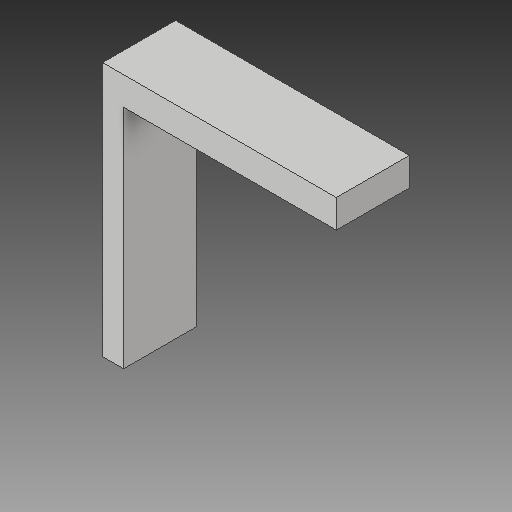
# Autodesk Inventor part: frame2
Saved by Autodesk Inventor 2019 (Build 230136000, 136)
## iProperties
Created: 2020-03-15
Part Number: frame2
Material: Generic
Document SubType Name: Modeling
Designer: Pulag
Mass: 4.15559 g
Surface Area: 27.541 cm^2
Volume: 4.15559 cm^3
Density: 1 g/cm^3
Appearance: Default
Author: Pulag
Autodesk Inventor part; units mm, degrees
ref_plane "YZ Plane" through (0, 0, 0) normal (1, 0, 0) x (0, 1, 0)
ref_plane "XZ Plane" through (0, 0, 0) normal (0, 1, 0) x (-1, 0, 0)
sketch "Sketch2" plane through (0, 0, 0) normal (0, 0, 1) x (1, 0, 0)
  line L0 (0.6059, 79.2071) -> (0.6059, 64.0071) projected
  line L1 (-21.8941, 64.0071) -> (-21.8941, 79.2071) projected
  line L2 (-35.7896, 30.0586) -> (-39.3896, 30.0586) projected
  line L3 (-39.3896, 25.2586) -> (-35.7896, 25.2586) projected
  line L4 (-35.7896, 25.2586) -> (-39.3896, 25.2586)
  line L5 (-39.3896, 25.2586) -> (-39.3896, 68.8314)
  line L6 (-35.7896, 64.0071) -> (-35.7896, 25.2586)
  line L7 (0.6059, 64.0071) -> (-35.7896, 64.0071)
  line L8 (-39.3896, 64.0071) -> (-39.3896, 68.8314)
  line L9 (-39.3896, 68.8314) -> (0.6059, 68.8314)
  line L10 (0.6059, 68.8314) -> (0.6059, 64.0071)
  point P0 (0, 0)
  constraints: 14 end point, 3 parallel, 2 horizontal, 2 perpendicular
ref_plane "Work Plane1" through (-26.6941, 57.0071, 12.5) normal (0, 0, 1) x (1, 0, 0)
extrude "Extrusion1" add sketch "Sketch2" along normal up to surface (12.5 mm away)
body "Solid1"
